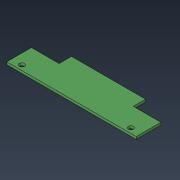
# Autodesk Inventor part: Ballsensor IR Platine
Saved by Autodesk Inventor 2022.1 (Build 261234020, 234B)
## iProperties
Part Number: Ballsensor IR Platine
Material: Phenolharz
Document SubType Name: Modeling
Designer: rYan
Mass: 0.924038 g
Surface Area: 14.8742 cm^2
Volume: 0.669593 cm^3
Density: 1.38 g/cm^3
Appearance: Glatt - waldgrün
Author: rYan
Autodesk Inventor part; units mm, degrees
ref_plane "YZ Plane" through (0, 0, 0) normal (1, 0, 0) x (0, 1, 0)
ref_plane "XZ Plane" through (0, 0, 0) normal (0, 1, 0) x (-1, 0, 0)
ref_plane "XY Plane" through (0, 0, 0) normal (0, 0, 1) x (1, 0, 0)
sketch "Skizze1" plane through (0, 0, 0) normal (0, 0, 1) x (1, 0, 0)
  line L0 (-15, 5) -> (15, 5)
  line L1 (15, 5) -> (15, 0)
  line L2 (-15, 0) -> (-15, 5)
  line L3 (26.2, 0) -> (26.2, -10)
  line L4 (26.2, -10) -> (-26.2, -10)
  line L5 (-26.2, -10) -> (-26.2, 0)
  line L6 (-26.2, 0) -> (-15, 0)
  line L7 (15, 0) -> (26.2, 0)
  line L8 (0, 8) -> (0, -13) projected
  point P0 (0, 0)
  dimension "d0" = 30
  dimension "d1" = 5
  dimension "d2" = 52.4
  dimension "d3" = 10
  constraints: 16 end point, 4 parallel, 3 horizontal, 3 perpendicular, 1 point on line, 3 other
  measures "d0" distance of L0.start L0.end
  measures "d1" distance of L0.end L1.end
  measures "d2" distance of L3.end L4.end
  measures "d3" distance of L3.start L3.end
extrude "Extrusion1" add sketch "Skizze1" along normal blind 1
sketch "Skizze3" plane through (0, 0, 1) normal (0, 0, 1) x (1, 0, 0)
  line L0 (0, 8) -> (0, -13) projected
  line L1 (-36.68, 0) -> (36.68, 0) projected
  point P0 (0, 0)
  point P1 (22.05, -8)
  point P2 (-22.05, -8)
  dimension "d18" = 22.05
  dimension "d19" = 8
  constraints: 1 symmetric about line
  measures "d18" distance from line of point (22.05, -8) L0
  measures "d19" distance from line of L1 point (-22.05, -8)
hole "Bohrung2" at (22.05, -8, 1) at (-22.05, -8, 1) direction (0, 0, -1) diameter 2.1 end through all
sketch "Skizze4" plane through (0, 0, 0) normal (0, 0, -1) x (-1, 0, 0)
  line L0 (-2.05, 4.6) -> (-3.45, 4.6)
  line L1 (-3.45, 4.6) -> (-3.45, 1.6)
  line L2 (-3.45, 1.6) -> (-2.05, 1.6)
  line L3 (-2.05, 1.6) -> (-2.05, 4.6)
  line L4 (15, 5) -> (-15, 5) projected
  line L5 (0, -13) -> (0, 8) projected
  line L6 (-2.75, 4.6) -> (-2.75, 1.6) construction
  point P0 (0, 0)
  dimension "d27" = 1.4
  dimension "d28" = 0.4
  dimension "d29" = 3
  dimension "d31" = 2.75
  constraints: 10 end point, 2 midpoint, 2 parallel, 1 horizontal, 1 perpendicular
  measures "d27" distance of L0.start L0.end
  measures "d28" distance between parallel lines of L4 L0
  measures "d29" distance of L2.end L0.start
  measures "d31" distance between parallel lines of L6 L5
extrude "Extrusion2" add sketch "Skizze4" along normal blind 0.05
pattern_linear "Rechteckige Anordnung2" count 6 spacing 2 along (1, 0, 0) of "Extrusion2"
mirror "Spiegeln2" about plane through (0, 0, 0) normal (1, 0, 0) of "Extrusion2", "Rechteckige Anordnung2"
